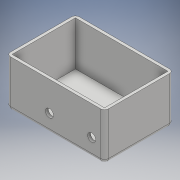
# Autodesk Inventor part: relay-housing
Saved by Autodesk Inventor 2018 (Build 220112000, 112)
## iProperties
Created: 2018-03-19
Part Number: relay-housing
Material: Generic
Document SubType Name: Modeling
Designer: matth
Density: 1 g/cm^3
Appearance: Default
Author: matth
Autodesk Inventor part; units mm, degrees
ref_plane "YZ Plane" through (0, 0, 0) normal (1, 0, 0) x (0, 1, 0)
ref_plane "XZ Plane" through (0, 0, 0) normal (0, 1, 0) x (-1, 0, 0)
ref_plane "XY Plane" through (0, 0, 0) normal (0, 0, 1) x (1, 0, 0)
sketch "Sketch1" plane through (0, 0, 0) normal (0, 0, 1) x (1, 0, 0)
  line L0 (0, 0) -> (46, 0)
  line L1 (46, 0) -> (46, 31.5)
  line L2 (46, 31.5) -> (0, 31.5)
  line L3 (0, 31.5) -> (0, 0)
  line L4 (-1.4, 32.9) -> (47.4, 32.9)
  line L5 (47.4, 32.9) -> (47.4, -1.4)
  line L6 (47.4, -1.4) -> (-1.4, -1.4)
  line L7 (-1.4, -1.4) -> (-1.4, 32.9)
  dimension "d0" = 46
  dimension "d1" = 31.5
  dimension "d2" = 1.4
  constraints: 16 end point, 4 parallel, 2 perpendicular, 1 horizontal, 3 other
  measures "d0" distance of L2.end L1.end
  measures "d1" distance of L1.end L0.end
  measures "d2" distance between parallel lines of L2 L4
extrude "Extrusion1" add sketch "Sketch1" along normal blind 22
sketch "Sketch2" plane through (0, 0, 0) normal (0, 0, -1) x (-1, 0, 0)
  line L0 (1.4, -1.4) -> (1.4, 32.9) projected
  line L1 (-47.4, -1.4) -> (1.4, -1.4) projected
  line L2 (1.4, 32.9) -> (-47.4, 32.9) projected
  line L3 (-47.4, 32.9) -> (-47.4, -1.4) projected
  point P0 (0, 0)
extrude "Extrusion2" add sketch "Sketch2" along normal blind 1.4
sketch "Sketch3" plane through (-1.4, -1.4, 22) normal (0, -1, 0) x (1, 0, 0)
  circle A0 centre (21.4, -14.5673) radius 2
  line L0 (1.4, -22) -> (1.4, 0) projected
  circle A1 centre (42.4, -14.5673) radius 2
  line L1 (47.4, -22) -> (47.4, 0) projected
  dimension "d7" = 4
  dimension "d8" = 20
  dimension "d9" = 4
  dimension "d10" = 5
  constraints: 2 centre point
  measures "d7" diameter of A0
  measures "d8" distance from line of L0 A0.centre
  measures "d9" diameter of A1
  measures "d10" distance from line of L1 A1.centre
extrude "Extrusion3" cut sketch "Sketch3" against normal blind 1.4
fillet "Fillet1" radius 2 8 edges at (-1.4, -1.4, 10.3) (47.4, -1.4, 10.3) (47.4, 32.9, 10.3) (-1.4, 32.9, 10.3) (47.4, 15.75, -1.4) (23, -1.4, -1.4) (-1.4, 15.75, -1.4) (23, 32.9, -1.4)
body "Solid1"
